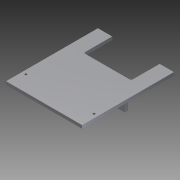
# Autodesk Inventor part: LIDAR Bracket
Saved by Autodesk Inventor 2012 (Build 160160000, 160)
## iProperties
Created: 2012-05-12
Part Number: LIDAR Bracket
Material: Default
Document SubType Name: Modeling
Designer: esv
Density: 1 g/cm^3
Author: esv
Autodesk Inventor part; units mm, degrees
ref_plane "YZ Plane" through (0, 0, 0) normal (1, 0, 0) x (0, 1, 0)
ref_plane "XZ Plane" through (0, 0, 0) normal (0, 1, 0) x (-1, 0, 0)
ref_plane "XY Plane" through (0, 0, 0) normal (0, 0, 1) x (1, 0, 0)
sketch "Sketch1" plane through (0, 0, 0) normal (0, 0, 1) x (1, 0, 0)
  line L0 (0, 0) -> (101.6, 0)
  line L1 (101.6, 0) -> (101.6, 40)
  line L2 (101.6, 40) -> (0, 40)
  line L3 (0, 40) -> (0, 0)
  dimension "d0" = 101.6
  dimension "d1" = 40
  constraints: 8 end point, 2 parallel, 1 horizontal, 1 perpendicular
  measures "d0" distance of L0.start L0.end
  measures "d1" distance of L2.end L0.start
extrude "Mounting Plate" add sketch "Sketch1" along normal blind 6.35
sketch "Sketch2" plane through (0, 40, 0) normal (0, 1, 0) x (1, 0, 0)
  line L0 (0, -6.35) -> (101.6, -6.35) projected
  line L1 (101.6, 0) -> (101.6, -6.35) projected
  line L2 (101.6, 0) -> (0, 0) projected
  line L3 (0, 0) -> (0, -6.35) projected
  line L4 (-25.4, 66.675) -> (127, 66.675)
  line L5 (127, 66.675) -> (127, -117.475)
  line L6 (127, -117.475) -> (-25.4, -117.475)
  line L7 (-25.4, -117.475) -> (-25.4, 66.675)
  line L8 (3.175, 66.675) -> (98.425, 66.675)
  line L9 (98.425, 66.675) -> (98.425, 12.7)
  line L10 (95.25, 9.525) -> (6.35, 9.525)
  line L11 (3.175, 12.7) -> (3.175, 66.675)
  arc A0 (3.175, 12.7) -> (6.35, 9.525) centre (6.35, 12.7) ccw
  arc A1 (95.25, 9.525) -> (98.425, 12.7) centre (95.25, 12.7) ccw
  point P0 (98.425, 9.525)
  point P1 (3.175, 9.525)
  point P2 (50.8, 66.675)
  point P3 (50.8, 0)
  point P4 (50.8, 9.525)
  dimension "d4" = 152.4
  dimension "d5" = 184.15
  dimension "d6" = 95.25
  dimension "d7" = 57.15
  dimension "d8" = 9.525
  dimension "d9" = 3.175
  constraints: 16 end point, 5 point on line, 4 midpoint, 4 parallel, 4 point on circle, 4 tangent, 2 centre point, 2 horizontal, 2 perpendicular, 1 equal radius, 1 vertical alignment
  measures "d4" distance of L5.end L6.end
  measures "d5" distance of L4.end L5.end
  measures "d6" distance of point (98.425, 9.525) point (3.175, 9.525)
  measures "d7" distance between parallel lines of L4 L10
  measures "d8" distance between parallel lines of L2 L10
  measures "d9" radius of A0
extrude "Back Plate" add sketch "Sketch2" along normal blind 6.35 contours L3 L2 L1 L0 | L4 L11 A0 L10 A1 L9 L5 L6 L7
sketch "Sketch3" plane through (0, 0, 0) normal (0, 0, -1) x (-1, 0, 0)
  line L0 (0, 0) -> (-101.6, 0) projected
  line L1 (-101.6, 0) -> (-101.6, 40) projected
  line L2 (-88.9, 20) -> (-12.7, 20)
  line L3 (-6.35, 40) -> (-95.25, 40) projected
  point P0 (-50.8, 20)
  point P1 (-50.8, 40)
  dimension "d12" = 76.2
  dimension "d13" = 20
  constraints: 2 end point, 2 midpoint, 1 perpendicular, 1 vertical alignment
  measures "d12" distance of L2.start L2.end
  measures "d13" distance between parallel lines of L2 L0
hole "Hole1" at (88.9, 20, 0) at (12.7, 20, 0) direction (0, 0, 1) diameter 8.9916 end through all clearance for "Flat Head Machine Screw" size "M8" standard "Ansi Metric M Profile"
sketch "Sketch4" plane through (0, 40, 0) normal (0, -1, 0) x (1, 0, 0)
  line L0 (-25.4, 117.475) -> (127, 117.475) projected
  line L1 (0, 6.35) -> (101.6, 6.35) projected
  line L2 (-17.6, 85.725) -> (119.2, 85.725)
  point P0 (50.8, 85.725)
  point P1 (50.8, 117.475)
  dimension "d21" = 136.8
  dimension "d22" = 31.75
  constraints: 2 end point, 2 midpoint, 1 parallel, 1 vertical alignment
  measures "d21" distance of L2.start L2.end
  measures "d22" distance between parallel lines of L0 L2
hole "Hole2" at (-17.6, 40, 85.725) at (119.2, 40, 85.725) direction (0, 1, 0) diameter 4.4958 end through all clearance for "Flat Head Machine Screw" size "M4" standard "Ansi Metric M Profile"
body "Solid1"
